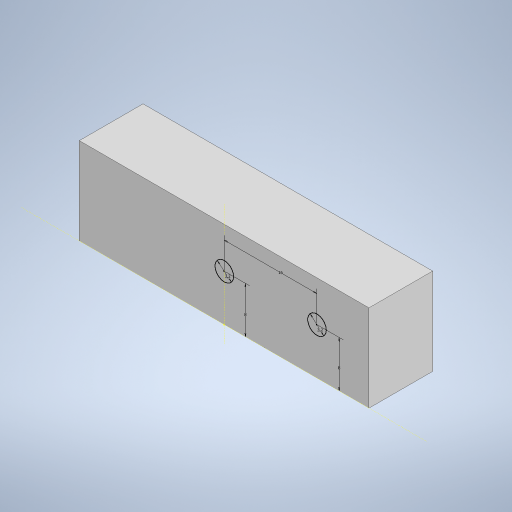
# Autodesk Inventor part: uMule-podpurka_elektronika
Saved by Autodesk Inventor 2024.2 (Build 282272000, 272)
## iProperties
Created: 2024-11-03
Part Number: uMule-podpurka_elektronika
Material: Ogólny
Document SubType Name: Modeling
Designer: owozn
Density: 1 g/cm^3
Appearance: Domyślna
Author: owozn
Autodesk Inventor part; units mm, degrees
ref_plane "YZ Plane" through (0, 0, 0) normal (1, 0, 0) x (0, 1, 0)
ref_plane "XZ Plane" through (0, 0, 0) normal (0, 1, 0) x (-1, 0, 0)
ref_plane "XY Plane" through (0, 0, 0) normal (0, 0, 1) x (1, 0, 0)
sketch "Szkic1" plane through (0, 0, 0) normal (0, 1, 0) x (-1, 0, 0)
  line L0 (0, -7.7) -> (0, 7.7) construction
  line L1 (35, 0) -> (-35, 0) construction
  line L2 (-25, 5.5) -> (25, 5.5)
  line L3 (25, 5.5) -> (25, -5.5)
  line L4 (25, -5.5) -> (-25, -5.5)
  line L5 (-25, -5.5) -> (-25, 5.5)
  line L6 (-25, 5.5) -> (25, -5.5) construction
  line L7 (25, 5.5) -> (-25, -5.5) construction
  point P0 (0, 0)
  dimension "d0" = 50
  dimension "d1" = 11
  constraints: 12 end point, 2 midpoint, 2 parallel, 1 horizontal, 1 perpendicular
  measures "d0" distance of L3.end L4.end
  measures "d1" distance of L2.end L3.end
extrude "Wyciągnięcie proste1" add sketch "Szkic1" along normal blind 15
sketch "Szkic2" plane through (-25, 0, 5.5) normal (0, 0, 1) x (1, 0, 0)
  line L0 (-10, 0) -> (60, 0) construction
  line L1 (25, -3) -> (25, 18) construction
  circle A0 centre (25, 8) radius 1.6
  circle A1 centre (41, 8) radius 1.6
  point P0 (25, 0)
  dimension "d4" = 3.2
  dimension "d5" = 3.2
  dimension "d6" = 8
  dimension "d7" = 8
  dimension "d8" = 16
  constraints: 2 centre point, 1 point on line
  measures "d4" diameter of A0
  measures "d5" diameter of A1
  measures "d6" distance from line of L0 A0.centre
  measures "d7" distance from line of L0 A1.centre
  measures "d8" distance of A1.centre A0.centre
